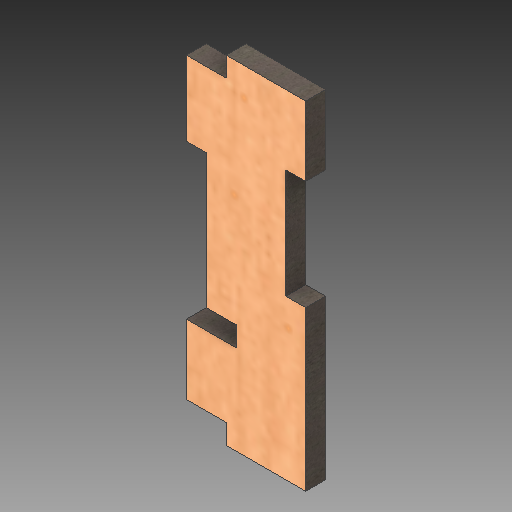
# Autodesk Inventor part: batTop
Saved by Autodesk Inventor 2019 (Build 230136000, 136)
## iProperties
Created: 2020-12-06
Part Number: batTop
Material: Дерево (береза)
Document SubType Name: Modeling
Designer: Professional
Density: 0.55 g/cm^3
Appearance: Береза — натуральный — полированный
Author: Professional
Autodesk Inventor part; units mm, degrees
ref_plane "YZ Plane" through (0, 0, 0) normal (1, 0, 0) x (0, 1, 0)
ref_plane "XZ Plane" through (0, 0, 0) normal (0, 1, 0) x (-1, 0, 0)
ref_plane "XY Plane" through (0, 0, 0) normal (0, 0, 1) x (1, 0, 0)
sketch "Эскиз1" plane through (0, 0, 0) normal (0, 0, 1) x (1, 0, 0)
  line L0 (-12, -16) -> (-12, -30)
  line L1 (-12, -30) -> (-4, -30)
  line L2 (-4, -34) -> (12, -34)
  line L3 (12, -34) -> (12, -2)
  line L4 (-8, 0) -> (8, 0)
  line L5 (-4, -30) -> (-4, -34)
  line L6 (-12, 30) -> (-4, 30)
  line L7 (-4, 34) -> (12, 34)
  line L8 (-4, 30) -> (-4, 34)
  line L9 (12, 34) -> (12, 20)
  line L10 (12, 20) -> (8, 20)
  line L11 (8, 20) -> (8, -2)
  line L12 (8, -2) -> (12, -2)
  line L13 (-8, -12) -> (-8, 15)
  line L14 (-8, 15) -> (-12, 15)
  line L15 (-12, 15) -> (-12, 30)
  line L16 (-8, -12) -> (-2, -12)
  line L17 (-2, -12) -> (-2, -16)
  line L18 (-2, -16) -> (-12, -16)
  point P0 (0, 0)
  point P1 (0, 0)
  dimension "d0" = 16
  dimension "d1" = 8
  dimension "d12" = 60
  dimension "d17" = 22
  dimension "d18" = 14
  dimension "d19" = 27
  dimension "d20" = 10
  dimension "d21" = 4
  dimension "d22" = 15
  constraints: 41 end point, 8 perpendicular, 4 horizontal, 4 symmetric about line, 4 vertical, 3 equal length, 2 point on line, 1 coincident, 1 midpoint
  measures "d0" distance of L2.end L2.start
  measures "d1" distance of L0.end L1.end
  measures "d12" distance between parallel lines of L6 L1
  measures "d17" distance from line of L10 L11.end
  measures "d18" distance between parallel lines of L7 L10
  measures "d19" distance of L13.start L13.end
  measures "d20" distance of L17.end L0.start
  measures "d21" distance of L16.end L17.end
  measures "d22" distance from line of L14 L4.start
extrude "Выдавливание1" add sketch "Эскиз1" along normal blind 4
